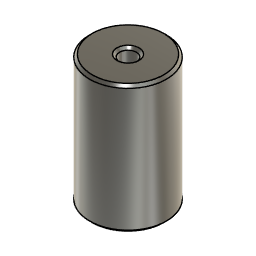
Test Standoff v5 (Autodesk Fusion 360 design; units mm, degrees)
Autodesk Fusion 360 part; units mm, degrees
sketch "Sketch1" plane through (0, 0, 0) normal (0, 0, 1) x (1, 0, 0)
  circle A0 centre (0, 0) radius 1.65
  circle A1 centre (0, 0) radius 7.5
  dimension "d1" = 3.3
  dimension "d2" = 15
  constraint coincident A0.centre A1.centre
  measures "d1" diameter of A0
  measures "d2" diameter of A1
extrude "Extrude1" add sketch "Sketch1" along normal blind 25
chamfer "Chamfer1" distance 0.5 angle 45 2 faces at (5.5159, -0.4546, 25) (5.5159, -0.4546, 0)
